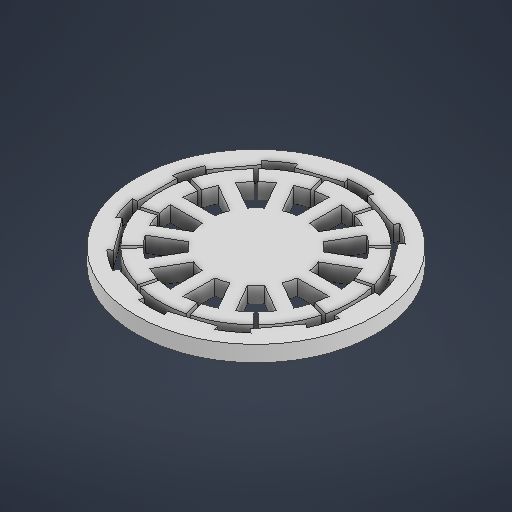
# Autodesk Inventor part: RotorEstatorA
Saved by Autodesk Inventor 2025.1 (Build 291241020, 241B)
## iProperties
Created: 2024-11-08
Part Number: RotorEstatorA
Material: Generic
Document SubType Name: Modeling
Designer: gusta
Density: 1 g/cm^3
Appearance: Default
Author: gusta
Autodesk Inventor part; units mm, degrees
ref_plane "YZ Plane" through (0, 0, 0) normal (1, 0, 0) x (0, 1, 0)
ref_plane "XZ Plane" through (0, 0, 0) normal (0, 1, 0) x (-1, 0, 0)
ref_plane "XY Plane" through (0, 0, 0) normal (0, 0, 1) x (1, 0, 0)
sketch "Sketch1" plane through (0, 0, 0) normal (0, 1, 0) x (-1, 0, 0)
  circle A0 centre (0, 0) radius 75
  line L0 (0, -75) -> (0, -65)
  circle A1 centre (0, 0) radius 65 construction
  line L1 (65, 0) -> (62, 0) construction
  line L2 (65, 0) -> (65, -12.5) construction
  line L3 (65, -12.5) -> (62, -12.5)
  line L4 (62, -12.5) -> (62, 0)
  line L5 (65, 0) -> (65, 12.5) construction
  line L6 (65, 12.5) -> (62, 12.5)
  line L7 (62, 12.5) -> (62, 0)
  circle A2 centre (0, 0) radius 66.191
  line L8 (57.5064, 26.33) -> (50.1591, 36.4427)
  line L9 (42.8117, 46.5554) -> (50.1591, 36.4427)
  line L10 (59.9334, 28.0933) -> (57.5064, 26.33)
  line L11 (45.2388, 48.3188) -> (42.8117, 46.5554)
  line L12 (31.0473, 55.1028) -> (19.1591, 58.9655)
  line L13 (7.2708, 62.8282) -> (19.1591, 58.9655)
  line L14 (31.9743, 57.956) -> (31.0473, 55.1028)
  line L15 (8.1979, 65.6814) -> (7.2708, 62.8282)
  line L16 (-7.2708, 62.8282) -> (-19.1591, 58.9655)
  line L17 (-31.0473, 55.1028) -> (-19.1591, 58.9655)
  line L18 (-8.1979, 65.6814) -> (-7.2708, 62.8282)
  line L19 (-31.9743, 57.956) -> (-31.0473, 55.1028)
  line L20 (-42.8117, 46.5554) -> (-50.1591, 36.4427)
  line L21 (-57.5064, 26.33) -> (-50.1591, 36.4427)
  line L22 (-45.2388, 48.3188) -> (-42.8117, 46.5554)
  line L23 (-59.9334, 28.0933) -> (-57.5064, 26.33)
  line L24 (-62, 12.5) -> (-62, 0)
  line L25 (-62, -12.5) -> (-62, 0)
  line L26 (-65, 12.5) -> (-62, 12.5)
  line L27 (-65, -12.5) -> (-62, -12.5)
  line L28 (-57.5064, -26.33) -> (-50.1591, -36.4427)
  line L29 (-42.8117, -46.5554) -> (-50.1591, -36.4427)
  line L30 (-59.9334, -28.0933) -> (-57.5064, -26.33)
  line L31 (-45.2388, -48.3188) -> (-42.8117, -46.5554)
  line L32 (-31.0473, -55.1028) -> (-19.1591, -58.9655)
  line L33 (-7.2708, -62.8282) -> (-19.1591, -58.9655)
  line L34 (-31.9743, -57.956) -> (-31.0473, -55.1028)
  line L35 (-8.1979, -65.6814) -> (-7.2708, -62.8282)
  line L36 (7.2708, -62.8282) -> (19.1591, -58.9655)
  line L37 (31.0473, -55.1028) -> (19.1591, -58.9655)
  line L38 (8.1979, -65.6814) -> (7.2708, -62.8282)
  line L39 (31.9743, -57.956) -> (31.0473, -55.1028)
  line L40 (42.8117, -46.5554) -> (50.1591, -36.4427)
  line L41 (57.5064, -26.33) -> (50.1591, -36.4427)
  line L42 (45.2388, -48.3188) -> (42.8117, -46.5554)
  line L43 (59.9334, -28.0933) -> (57.5064, -26.33)
  dimension "d0" = 150
  dimension "d1" = 10
  dimension "d2" = 3
  dimension "d3" = 12.5
  dimension "d4" = 3
  dimension "d7" = 360
  constraints: 88 end point, 3 coincident, 2 point on circle, 2 symmetric about line, 2 vertical, 1 centre point, 1 horizontal, 1 perpendicular, 1 tangent, 1 vertical alignment, 96 other
  measures "d1" distance of L0.start L0.end
  measures "d2" distance of L1.start L1.end
  measures "d3" distance of L1.start L2.end
  measures "d4" distance of L2.end L3.end
extrude "Extrusion1" add sketch "Sketch1" along normal blind 10 contours A0 | L3 L4 L7 L6 A2 | A2 L42 L40 L41 L43 | A2 L38 L36 L37 L39 | L10 L8 L9 L11 A2 | L14 L12 L13 L15 A2 | A2 L34 L32 L33 L35 | L18 L16 L17 L19 A2 | A2 L30 L28 L29 L31 | L22 L20 L21 L23 A2 | A2 L26 L24 L25 L27
sketch "Sketch2" plane through (0, 10, 0) normal (0, 1, 0) x (1, 0, 0)
  circle A0 centre (0, 0) radius 30
  line L0 (-62, -12.5) -> (-62, 12.5) projected
  line L1 (-62, 0) -> (-60, 0)
  arc A1 (-58.2177, 14.5153) -> (-60, 0) centre (0, 0) ccw
  line L2 (0, 0) -> (-58.2177, 14.5153) construction
  line L3 (0, 0) -> (-60, 0) construction
  line L4 (-60, 0) -> (-50, 0)
  arc A2 (-48.5148, 12.0961) -> (-50, 0) centre (0, 0) ccw
  line L5 (-58.2177, 14.5153) -> (-48.5148, 12.0961)
  arc A3 (-60, 0) -> (-58.2177, -14.5153) centre (0, 0) ccw
  arc A4 (-50, 0) -> (-48.5148, -12.0961) centre (0, 0) ccw
  line L6 (-58.2177, -14.5153) -> (-48.5148, -12.0961)
  line L7 (-50, 0) -> (-50, 4)
  line L8 (-50, 4) -> (-0.1794, 4)
  line L9 (-50, -4) -> (-0.1794, -4)
  arc A5 (-57.6757, -16.5382) -> (-51.9615, -30) centre (0, 0) ccw
  arc A6 (-51.9615, -30) -> (-43.1604, -41.6795) centre (0, 0) ccw
  line L10 (-43.1604, -41.6795) -> (-35.967, -34.7329)
  arc A7 (-43.3013, -25) -> (-35.967, -34.7329) centre (0, 0) ccw
  line L11 (-41.3013, -28.4641) -> (1.8447, -3.5538)
  line L12 (-45.3013, -21.5359) -> (-2.1553, 3.3744)
  arc A8 (-48.0631, -13.7819) -> (-43.3013, -25) centre (0, 0) ccw
  line L13 (-57.6757, -16.5382) -> (-48.0631, -13.7819)
  arc A9 (-41.6795, -43.1604) -> (-30, -51.9615) centre (0, 0) ccw
  arc A10 (-30, -51.9615) -> (-16.5382, -57.6757) centre (0, 0) ccw
  line L14 (-16.5382, -57.6757) -> (-13.7819, -48.0631)
  arc A11 (-25, -43.3013) -> (-13.7819, -48.0631) centre (0, 0) ccw
  line L15 (-21.5359, -45.3013) -> (3.3744, -2.1553)
  line L16 (-28.4641, -41.3013) -> (-3.5538, 1.8447)
  arc A12 (-34.7329, -35.967) -> (-25, -43.3013) centre (0, 0) ccw
  line L17 (-41.6795, -43.1604) -> (-34.7329, -35.967)
  arc A13 (-14.5153, -58.2177) -> (0, -60) centre (0, 0) ccw
  arc A14 (0, -60) -> (14.5153, -58.2177) centre (0, 0) ccw
  line L18 (14.5153, -58.2177) -> (12.0961, -48.5148)
  arc A15 (0, -50) -> (12.0961, -48.5148) centre (0, 0) ccw
  line L19 (4, -50) -> (4, -0.1794)
  line L20 (-4, -50) -> (-4, -0.1794)
  arc A16 (-12.0961, -48.5148) -> (0, -50) centre (0, 0) ccw
  line L21 (-14.5153, -58.2177) -> (-12.0961, -48.5148)
  arc A17 (16.5382, -57.6757) -> (30, -51.9615) centre (0, 0) ccw
  arc A18 (30, -51.9615) -> (41.6795, -43.1604) centre (0, 0) ccw
  line L22 (41.6795, -43.1604) -> (34.7329, -35.967)
  arc A19 (25, -43.3013) -> (34.7329, -35.967) centre (0, 0) ccw
  line L23 (28.4641, -41.3013) -> (3.5538, 1.8447)
  line L24 (21.5359, -45.3013) -> (-3.3744, -2.1553)
  arc A20 (13.7819, -48.0631) -> (25, -43.3013) centre (0, 0) ccw
  line L25 (16.5382, -57.6757) -> (13.7819, -48.0631)
  arc A21 (43.1604, -41.6795) -> (51.9615, -30) centre (0, 0) ccw
  arc A22 (51.9615, -30) -> (57.6757, -16.5382) centre (0, 0) ccw
  line L26 (57.6757, -16.5382) -> (48.0631, -13.7819)
  arc A23 (43.3013, -25) -> (48.0631, -13.7819) centre (0, 0) ccw
  line L27 (45.3013, -21.5359) -> (2.1553, 3.3744)
  line L28 (41.3013, -28.4641) -> (-1.8447, -3.5538)
  arc A24 (35.967, -34.7329) -> (43.3013, -25) centre (0, 0) ccw
  line L29 (43.1604, -41.6795) -> (35.967, -34.7329)
  arc A25 (58.2177, -14.5153) -> (60, 0) centre (0, 0) ccw
  arc A26 (60, 0) -> (58.2177, 14.5153) centre (0, 0) ccw
  line L30 (58.2177, 14.5153) -> (48.5148, 12.0961)
  arc A27 (50, 0) -> (48.5148, 12.0961) centre (0, 0) ccw
  line L31 (50, 4) -> (0.1794, 4)
  line L32 (50, -4) -> (0.1794, -4)
  arc A28 (48.5148, -12.0961) -> (50, 0) centre (0, 0) ccw
  line L33 (58.2177, -14.5153) -> (48.5148, -12.0961)
  arc A29 (57.6757, 16.5382) -> (51.9615, 30) centre (0, 0) ccw
  arc A30 (51.9615, 30) -> (43.1604, 41.6795) centre (0, 0) ccw
  line L34 (43.1604, 41.6795) -> (35.967, 34.7329)
  arc A31 (43.3013, 25) -> (35.967, 34.7329) centre (0, 0) ccw
  line L35 (41.3013, 28.4641) -> (-1.8447, 3.5538)
  line L36 (45.3013, 21.5359) -> (2.1553, -3.3744)
  arc A32 (48.0631, 13.7819) -> (43.3013, 25) centre (0, 0) ccw
  line L37 (57.6757, 16.5382) -> (48.0631, 13.7819)
  arc A33 (41.6795, 43.1604) -> (30, 51.9615) centre (0, 0) ccw
  arc A34 (30, 51.9615) -> (16.5382, 57.6757) centre (0, 0) ccw
  line L38 (16.5382, 57.6757) -> (13.7819, 48.0631)
  arc A35 (25, 43.3013) -> (13.7819, 48.0631) centre (0, 0) ccw
  line L39 (21.5359, 45.3013) -> (-3.3744, 2.1553)
  line L40 (28.4641, 41.3013) -> (3.5538, -1.8447)
  arc A36 (34.7329, 35.967) -> (25, 43.3013) centre (0, 0) ccw
  line L41 (41.6795, 43.1604) -> (34.7329, 35.967)
  arc A37 (14.5153, 58.2177) -> (0, 60) centre (0, 0) ccw
  arc A38 (0, 60) -> (-14.5153, 58.2177) centre (0, 0) ccw
  line L42 (-14.5153, 58.2177) -> (-12.0961, 48.5148)
  arc A39 (0, 50) -> (-12.0961, 48.5148) centre (0, 0) ccw
  line L43 (-4, 50) -> (-4, 0.1794)
  line L44 (4, 50) -> (4, 0.1794)
  arc A40 (12.0961, 48.5148) -> (0, 50) centre (0, 0) ccw
  line L45 (14.5153, 58.2177) -> (12.0961, 48.5148)
  arc A41 (-16.5382, 57.6757) -> (-30, 51.9615) centre (0, 0) ccw
  arc A42 (-30, 51.9615) -> (-41.6795, 43.1604) centre (0, 0) ccw
  line L46 (-41.6795, 43.1604) -> (-34.7329, 35.967)
  arc A43 (-25, 43.3013) -> (-34.7329, 35.967) centre (0, 0) ccw
  line L47 (-28.4641, 41.3013) -> (-3.5538, -1.8447)
  line L48 (-21.5359, 45.3013) -> (3.3744, 2.1553)
  arc A44 (-13.7819, 48.0631) -> (-25, 43.3013) centre (0, 0) ccw
  line L49 (-16.5382, 57.6757) -> (-13.7819, 48.0631)
  arc A45 (-43.1604, 41.6795) -> (-51.9615, 30) centre (0, 0) ccw
  arc A46 (-51.9615, 30) -> (-57.6757, 16.5382) centre (0, 0) ccw
  line L50 (-57.6757, 16.5382) -> (-48.0631, 13.7819)
  arc A47 (-43.3013, 25) -> (-48.0631, 13.7819) centre (0, 0) ccw
  line L51 (-45.3013, 21.5359) -> (-2.1553, -3.3744)
  line L52 (-41.3013, 28.4641) -> (1.8447, 3.5538)
  arc A48 (-35.967, 34.7329) -> (-43.3013, 25) centre (0, 0) ccw
  line L53 (-43.1604, 41.6795) -> (-35.967, 34.7329)
  point P0 (-23.7488, -18.3302)
  point P1 (-18.3302, -23.7488)
  point P2 (-28.384, -41.1625)
  point P3 (-21.4558, -45.1625)
  point P4 (-11.402, -27.7488)
  point P5 (-4, -29.7321)
  point P6 (-4, -49.8397)
  point P7 (4, -49.8397)
  point P8 (4, -29.7321)
  point P9 (11.402, -27.7488)
  point P10 (21.4558, -45.1625)
  point P11 (28.384, -41.1625)
  point P12 (18.3302, -23.7488)
  point P13 (23.7488, -18.3302)
  point P14 (41.1625, -28.384)
  point P15 (45.1625, -21.4558)
  point P16 (27.7488, -11.402)
  point P17 (29.7321, -4)
  point P18 (49.8397, -4)
  point P19 (49.8397, 4)
  point P20 (29.7321, 4)
  point P21 (27.7488, 11.402)
  point P22 (45.1625, 21.4558)
  point P23 (41.1625, 28.384)
  point P24 (23.7488, 18.3302)
  point P25 (18.3302, 23.7488)
  point P26 (28.384, 41.1625)
  point P27 (21.4558, 45.1625)
  point P28 (11.402, 27.7488)
  point P29 (4, 29.7321)
  point P30 (4, 49.8397)
  point P31 (-4, 49.8397)
  point P32 (-4, 29.7321)
  point P33 (-11.402, 27.7488)
  point P34 (-21.4558, 45.1625)
  point P35 (-28.384, 41.1625)
  point P36 (-18.3302, 23.7488)
  point P37 (-23.7488, 18.3302)
  point P38 (-41.1625, 28.384)
  point P39 (-45.1625, 21.4558)
  point P40 (-27.7488, 11.402)
  point P41 (-29.7321, 4)
  point P42 (-49.8397, 4)
  point P43 (-49.8397, -4)
  point P44 (-29.7321, -4)
  point P45 (-27.7488, -11.402)
  point P46 (-45.1625, -21.4558)
  point P47 (-41.1625, -28.384)
  dimension "d11" = 60
  dimension "d12" = 2
  dimension "d13" = 14
  dimension "d14" = 10
  dimension "d15" = 4
  dimension "d18" = 360
  constraints: 106 end point, 96 point on circle, 48 centre point, 26 coincident, 4 symmetric about line, 2 horizontal, 2 point on line, 1 collinear, 1 midpoint, 1 tangent, 1 vertical, 245 other
  measures "d12" distance of L1.start L1.end
  measures "d13" angle of L2 L3
  measures "d14" distance of L1.end L4.end
  measures "d15" distance of L4.end L7.end
extrude "Extrusion2" add sketch "Sketch2" against normal blind 10 contours A0 L32 L27 L36 L31 | A0 L31 A27 A28 L32 | L31 L36 A0 | A0 L27 L32 | L36 L31 L40 L35 A0 | A0 L35 A31 A32 L36 | A27 L30 A26 A25 L33 A28 | L36 L27 L40 L31 | L27 A23 A24 L28 A0 | A0 L28 L23 L32 L27 | L32 L23 L36 L27 | L35 L40 A0 | A32 A31 L34 A30 A29 L37 | L40 L27 L44 L31 | L31 L44 L35 L40 | L36 L23 L40 L27 | A0 L23 L28 | A23 L26 A22 A21 L29 A24 | L32 L19 L36 L23 | L23 L28 L19 L32 | L40 L35 L44 L39 A0 | A0 L39 A35 A36 L40 | L44 L27 L48 L31 | L31 L48 L35 L44 | L40 L23 L44 L27 | L36 L19 L40 L23 | L23 A19 A20 L24 A0 | A0 L24 L19 L28 L23 | L32 L15 L36 L19 | L19 L28 L15 L32 | L39 L44 A0 | A36 A35 L38 A34 A33 L41 | L35 L48 L39 L44 | L48 L27 L44 L23 L40 L19 L36 L15 L32 L11 L28 L9 L24 L51 L20 L47 L16 L43 L12 L39 L8 L35 L52 L31 | L31 L52 L35 L48 | A0 L19 L24 | A19 L22 A18 A17 L25 A20 | L19 L24 L15 L28 | L15 L28 L11 L32 | L44 L39 L48 L43 A0 | A0 L43 A39 A40 L44 | L35 L52 L39 L48 | L19 A15 A16 L20 A0 | A0 L20 L15 L24 L19 | L15 L24 L11 L28 | L43 L48 A0 | A40 A39 L42 A38 A37 L45 | L39 L52 L43 L48 | L35 L8 L39 L52 | A0 L15 L20 | A15 L18 A14 A13 L21 A16 | L15 L20 L11 L24 | L11 L24 L9 L28 | L48 L43 L52 L47 A0 | A0 L47 A43 A44 L48 | L39 L8 L43 L52 | L15 A11 A12 L16 A0 | A0 L16 L11 L20 L15 | L11 L20 L9 L24 | L47 L52 A0 | A44 A43 L46 A42 A41 L49 | L43 L8 L47 L52 | L39 L12 L43 L8 | A0 L11 L16 | A11 L14 A10 A9 L17 A12 | L11 L16 L9 L20 | L9 L20 L51 L24 | L52 L47 L8 L51 A0 | A0 L51 A47 A48 L52 | L43 L12 L47 L8 | L11 A7 A8 L12 A0 | A0 L12 L9 L16 L11 | L9 L16 L51 L20 | L51 L8 A0 | A48 A47 L50 A46 A45 L53 | L47 L12 L51 L8 | L43 L16 L47 L12 | A0 L9 L12 | A7 L10 A6 A5 L13 A8 | L9 L12 L51 L16 | L51 L16 L47 L20 | L8 L51 L12 L9 A0 | A0 L9 A4 A2 L8 | L47 L16 L51 L12 | L8 L7 L4 A1 L5 A2 | A4 L6 A3 L4
thicken "Thicken1" operation add thickness 1 both sides no extend neighbours no toward (1, 0, 0) faces at (-50, 6.6667, -1.3333)
body "Solid1"
